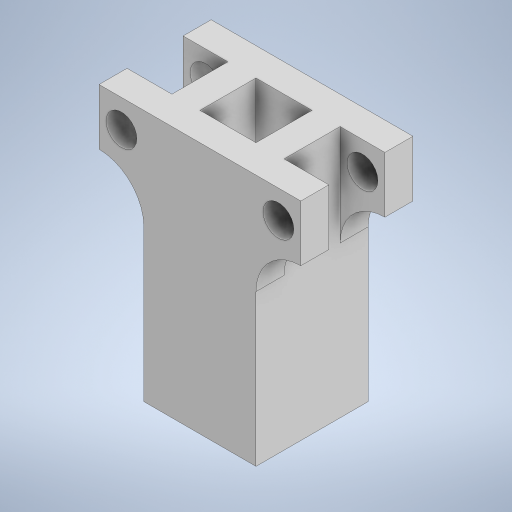
# Autodesk Inventor part: asta con serraggio pinza
Saved by Autodesk Inventor 2023 (Build 270158000, 158)
## iProperties
Created: 2023-08-20
Part Number: asta con serraggio pinza
Material: Generico
Document SubType Name: Sheet Metal
Designer: Admin
Density: 1 g/cm^3
Sheet Metal Rule: Default_mm
Appearance: Default
Author: Admin
Autodesk Inventor part; units mm, degrees
ref_plane "YZ Plane" through (0, 0, 0) normal (1, 0, 0) x (0, 1, 0)
ref_plane "XZ Plane" through (0, 0, 0) normal (0, 1, 0) x (-1, 0, 0)
ref_plane "XY Plane" through (0, 0, 0) normal (0, 0, 1) x (1, 0, 0)
sketch "Schizzo1" plane through (0, 0, 0) normal (0, 1, 0) x (-1, 0, 0)
  line L0 (5, 5) -> (-5, 5)
  line L1 (-5, 5) -> (-5, -5)
  line L2 (-5, -5) -> (5, -5)
  line L3 (5, -5) -> (5, 5)
  line L4 (10, 10) -> (-10, 10)
  line L5 (-10, 10) -> (-10, -10)
  line L6 (-10, -10) -> (10, -10)
  line L7 (10, -10) -> (10, 10)
  line L8 (0, 0) -> (14, 0) construction
  line L9 (0, 0) -> (0, -16.4941) construction
  line L10 (10, 10) -> (18, 10)
  line L11 (18, 10) -> (18, 5)
  line L12 (18, 5) -> (10, 5)
  line L13 (10, -10) -> (18, -10)
  line L14 (18, -10) -> (18, -5)
  line L15 (18, -5) -> (10, -5)
  line L16 (-10, 10) -> (-18, 10)
  line L17 (-18, 10) -> (-18, 5)
  line L18 (-18, 5) -> (-10, 5)
  line L19 (-10, -10) -> (-18, -10)
  line L20 (-18, -10) -> (-18, -5)
  line L21 (-18, -5) -> (-10, -5)
  dimension "d0" = 20
  dimension "d1" = 10
  dimension "d2" = 8
  dimension "d3" = 5
  constraints: 44 end point, 9 symmetric about line, 6 perpendicular, 4 horizontal, 4 parallel, 1 point on line, 1 vertical, 4 other
  measures "d0" distance of L6.end L4.start
  measures "d1" distance of L2.end L0.start
  measures "d2" distance of L4.start L10.end
  measures "d3" distance of L10.end L11.end
extrude "Estrusione1" add sketch "Schizzo1" along normal blind 10 and the other way blind 35 contours L7 L6 L5 L4
extrude "Estrusione2" add sketch "Schizzo1" along normal blind 10 contours L10 L11 L12 L7 | L5 L18 L17 L16 | L15 L14 L13 L7 | L5 L19 L20 L21
fillet "Raccordo1" radius 8 4 edges at (10, 0, 7.5) (10, 0, -7.5) (-10, 0, -7.5) (-10, 0, 7.5)
sketch "Schizzo2" plane through (0, 0, 0) normal (0, 0, 1) x (1, 0, 0)
  line L0 (-18, 0) -> (-18, 10) projected
  line L1 (-18, 10) -> (18, 10) projected
  line L2 (18, 0) -> (18, 10) projected
  arc A0 (18, 0) -> (10, -8) centre (18, -8) ccw projected
  arc A1 (-10, -8) -> (-18, 0) centre (-18, -8) ccw projected
  line L3 (-10, -8) -> (-10, 10) projected
  line L4 (10, 10) -> (10, -8) projected
  circle A2 centre (-14, 5) radius 2.75
  line L5 (0, 0) -> (0, 11.3165) construction
  circle A3 centre (14, 5) radius 2.75
  dimension "d11" = 5.5
  dimension "d12" = 5
  dimension "d13" = 4
  constraints: 2 centre point, 2 end point, 1 symmetric about line, 1 vertical, 1 other
  measures "d11" diameter of A2
  measures "d12" distance from line of L1 A2.centre
  measures "d13" distance from line of L0 A2.centre
extrude "Estrusione3" cut sketch "Schizzo2" along normal through all both and the other way through all contours A2 | A3
equation "\"RaggioPiega\" = Spessore"
equation "\"LarghezzaScaricoPiega\" = Spessore"
equation "\"ProfonditàScaricoPiega\" = 0.5 * Spessore"
equation "\"DimensioniScaricoAngolo\" = 4 * Spessore"
equation "\"ResiduoMinimo\" = 2 * Spessore"
equation "\"RaggioTransizione\" = RaggioPiega"
equation "\"Dimensione_raggio_Jacobi\" = RaggioPiega"
equation "\"DimensioneGioco\" = Spessore"
equation "\"Spessore\" = 0.5"
